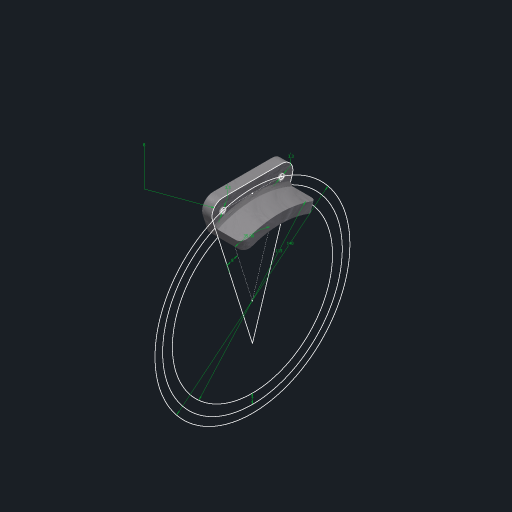
# Autodesk Inventor part: SEGURO_CANALETA
Saved by Autodesk Inventor 2024.3 (Build 283343000, 343)
## iProperties
Created: 2024-07-12
Part Number: SEGURO_CANALETA
Material: Steel, Mild, Welded
Document SubType Name: Modeling
Designer: Niler
Density: 7.85 g/cm^3
Appearance: Weld - Steel Mild
Author: Niler
Autodesk Inventor part; units mm, degrees
ref_plane "YZ Plane" through (0, 0, 0) normal (1, 0, 0) x (0, 1, 0)
ref_plane "XZ Plane" through (0, 0, 0) normal (0, 1, 0) x (-1, 0, 0)
ref_plane "XY Plane" through (0, 0, 0) normal (0, 0, 1) x (1, 0, 0)
sketch "Sketch1" plane through (0, 0, 0) normal (1, 0, 0) x (0, 1, 0)
  circle A0 centre (0, 0) radius 70
  line L0 (0, 0) -> (66.7602, 21.0494) construction
  line L1 (66.7602, -21.0494) -> (0, 0) construction
  line L2 (66.7602, -21.0494) -> (66.7602, 21.0494) construction
  circle A1 centre (66.7602, 21.0494) radius 1.65
  circle A2 centre (66.7602, -21.0494) radius 1.65
  circle A3 centre (0, 0) radius 57.5
  line L3 (64.3545, 28.6791) -> (-26.6041, 0)
  line L4 (-26.6041, 0) -> (64.3545, -28.6791)
  line L5 (74.7602, -21.0494) -> (74.7602, 21.0494)
  arc A4 (74.7602, 21.0494) -> (64.3545, 28.6791) centre (66.7602, 21.0494) ccw
  arc A5 (64.3545, -28.6791) -> (74.7602, -21.0494) centre (66.7602, -21.0494) ccw
  circle A6 centre (0, 0) radius 64.5
  point P0 (66.7602, 0)
  point P1 (51.8997, 24.7522)
  point P2 (51.8997, -24.7522)
  point P3 (58.6341, 26.8755)
  point P4 (58.6341, -26.8755)
  dimension "d0" = 140
  dimension "d1" = 35
  dimension "d2" = 3.3
  dimension "d3" = 3.3
  dimension "d4" = 115
  dimension "d5" = 8
  dimension "d6" = 8
  dimension "d7" = 7
  constraints: 12 end point, 7 centre point, 6 point on circle, 4 coincident, 4 tangent, 1 equal radius, 1 horizontal alignment, 1 midpoint, 1 vertical, 2 other
  measures "d0" diameter of A0
  measures "d1" angle of L0 L1
  measures "d2" diameter of A1
  measures "d3" diameter of A2
  measures "d4" diameter of A3
  measures "d5" distance between parallel lines of L0 L3
  measures "d6" radius of A4
  measures "d7" radial gap between concentric circles of A3 A6
extrude "Extrusion1" add sketch "Sketch1" against normal blind 7 contours A0 A2 L4 A6 L3 A1 | A0 A1 L3 A4 L5 A5 L4 A2 | A6 L4 A3 L3 picked at (61.9464, 3.0696)
extrude "Extrusion2" add sketch "Sketch1" along normal blind 20 contours A6 L4 A3 L3 picked at (61.9464, 3.0696)
fillet "Fillet1" radius 5 2 edges at (20, 55.2669, 25.8138) (20, 55.2669, -25.8138)
chamfer "Chamfer1" distance 2 angle 45 1 edges at (0, 64.5, 0)
sketch "Sketch2" plane through (0, 0, 0) normal (1, 0, 0) x (0, 0, -1)
  arc A0 (27.4814, 60.5559) -> (-27.4814, 60.5559) centre (0, 0) ccw projected
  line L0 (27.4814, 60.5559) -> (28.6791, 64.3545) projected
  arc A1 (28.6791, 64.3545) -> (21.0494, 74.7602) centre (21.0494, 66.7602) ccw projected
  line L1 (21.0494, 74.7602) -> (-21.0494, 74.7602) projected
  arc A2 (-21.0494, 74.7602) -> (-28.6791, 64.3545) centre (-21.0494, 66.7602) ccw projected
  line L2 (-28.6791, 64.3545) -> (-27.4814, 60.5559) projected
  circle A3 centre (-21.0494, 66.7602) radius 1.65 projected
  circle A4 centre (21.0494, 66.7602) radius 1.65 projected
  circle A5 centre (-21.0494, 66.7602) radius 2.9
  circle A6 centre (21.0494, 66.7602) radius 2.9
  dimension "d16" = 5.8
  dimension "d17" = 5.8
  constraints: 2 centre point, 2 coincident
  measures "d16" diameter of A5
  measures "d17" diameter of A6
extrude "Extrusion3" cut sketch "Sketch2" against normal blind 4 contours A3 | A4 | A5 | A6
body "Solid1"
